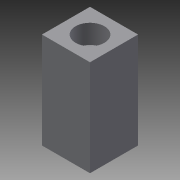
# Autodesk Inventor part: screw holder
Saved by Autodesk Inventor 2015 (Build 190159000, 159)
## iProperties
Created: 2018-04-13
Part Number: screw holder
Material: Generic
Document SubType Name: Modeling
Designer: Toby
Density: 1 g/cm^3
Appearance: Default
Author: Toby
Autodesk Inventor part; units mm, degrees
ref_plane "YZ Plane" through (0, 0, 0) normal (1, 0, 0) x (0, 1, 0)
ref_plane "XZ Plane" through (0, 0, 0) normal (0, 1, 0) x (-1, 0, 0)
ref_plane "XY Plane" through (0, 0, 0) normal (0, 0, 1) x (1, 0, 0)
sketch "Sketch1" plane through (0, 0, 0) normal (0, 0, 1) x (1, 0, 0)
  line L0 (-10.4011, 3.8235) -> (-5.4011, 3.8235)
  line L1 (-5.4011, 3.8235) -> (-5.4011, -1.1765)
  line L2 (-5.4011, -1.1765) -> (-10.4011, -1.1765)
  line L3 (-10.4011, -1.1765) -> (-10.4011, 3.8235)
  point P0 (0, 0)
  dimension "d0" = 5
  dimension "d1" = 5
  constraints: 8 end point, 2 parallel, 1 horizontal, 1 perpendicular
  measures "d0" distance of L2.end L0.start
  measures "d1" distance of L0.start L0.end
extrude "Extrusion1" add sketch "Sketch1" along normal blind 10
sketch "Sketch2" plane through (0, 0, 10) normal (0, 0, 1) x (1, 0, 0)
  line L0 (-10.4011, 3.8235) -> (-5.4011, 3.8235) projected
  point P0 (0, 0)
  point P1 (-7.9011, 1.3235)
  dimension "d4" = 2.5
  measures "d4" distance from line of L0 point (-7.901, 1.324)
hole "Hole1" at (-7.9011, 1.3235, 10) direction (0, 0, -1) diameter 3 depth 2 tip angle 118
body "Solid1"
